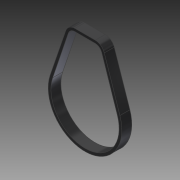
# Autodesk Inventor part: Weight Shifter Tension Strap 2
Saved by Autodesk Inventor 2014 SP1 (Build 180222100, 222)
## iProperties
Created: 2013-12-18
Part Number: Weight Shifter Tension Strap 2
Material: Rubber
Document SubType Name: Modeling
Designer: Moses
Density: 0.93 g/cm^3
Appearance: Rubber - Black - Version 1.1
Mass: 5.58759 g
Surface Area: 60.2332 cm^2
Volume: 6.00816 cm^3
Author: Moses
Autodesk Inventor part; units mm, degrees
ref_plane "YZ Plane" through (0, 0, 0) normal (1, 0, 0) x (0, 1, 0)
ref_plane "XZ Plane" through (0, 0, 0) normal (0, 1, 0) x (-1, 0, 0)
ref_plane "XY Plane" through (0, 0, 0) normal (0, 0, 1) x (1, 0, 0)
sketch "Sketch1" plane through (0, 0, 0) normal (0, 0, 1) x (1, 0, 0)
  line L0 (-15.875, 29.0994) -> (-12.7, 29.0994) construction
  line L1 (-15.875, 51.3244) -> (-15.875, 29.0994) construction
  arc A0 (-9.525, 57.6744) -> (-15.875, 51.3244) centre (-9.525, 51.3244) ccw construction
  line L2 (9.525, 57.6744) -> (-9.525, 57.6744) construction
  arc A1 (15.875, 51.3244) -> (9.525, 57.6744) centre (9.525, 51.3244) ccw construction
  line L3 (15.875, 29.0994) -> (15.875, 51.3244) construction
  line L4 (12.7, 29.0994) -> (15.875, 29.0994) construction
  line L5 (12.7, 51.3244) -> (12.7, 29.0994) construction
  arc A2 (12.7, 51.3244) -> (9.525, 54.4994) centre (9.525, 51.3244) ccw construction
  line L6 (-9.525, 54.4994) -> (9.525, 54.4994) construction
  arc A3 (-9.525, 54.4994) -> (-12.7, 51.3244) centre (-9.525, 51.3244) ccw construction
  line L7 (-12.7, 29.0994) -> (-12.7, 51.3244) construction
  line L8 (-30.0912, 10.1284) -> (-15.5432, 53.35)
  line L9 (30.0912, 10.1284) -> (15.5432, 53.35)
  arc A4 (-9.525, 57.6744) -> (-15.5432, 53.35) centre (-9.525, 51.3244) ccw
  arc A5 (15.5432, 53.35) -> (9.525, 57.6744) centre (9.525, 51.3244) ccw
  line L10 (-9.525, 57.6744) -> (9.525, 57.6744)
  arc A6 (-30.0912, 10.1284) -> (30.0912, 10.1284) centre (0, 0) ccw
  line L11 (-17.9505, 54.1603) -> (-32.4985, 10.9386)
  arc A7 (-32.4985, 10.9386) -> (32.4985, 10.9386) centre (0, 0) ccw
  line L12 (32.4985, 10.9386) -> (17.9505, 54.1603)
  arc A8 (17.9505, 54.1603) -> (9.525, 60.2144) centre (9.525, 51.3244) ccw
  line L13 (9.525, 60.2144) -> (-9.525, 60.2144)
  arc A9 (-9.525, 60.2144) -> (-17.9505, 54.1603) centre (-9.525, 51.3244) ccw
  circle A10 centre (0, 0) radius 31.75 construction
  dimension "d0" = 2.54
  constraints: 16 point on circle, 12 end point, 10 tangent, 6 centre point, 2 concentric, 1 coincident, 1 horizontal, 5 other
  measures "d0" distance between parallel lines of L13 L10
extrude "Extrusion1" add sketch "Sketch1" along normal blind 9.297
body "Solid1"
